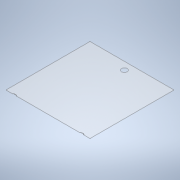
# Autodesk Inventor part: porta
Saved by Autodesk Inventor 2022 (Build 260153000, 153)
## iProperties
Created: 2022-02-18
Part Number: porta
Material: Acrílico
Document SubType Name: Modeling
Designer: mathe
Density: 1.188 g/cm^3
Appearance: Transparente - Claro
Author: mathe
Autodesk Inventor part; units mm, degrees
ref_plane "YZ Plane" through (0, 0, 0) normal (1, 0, 0) x (0, 1, 0)
ref_plane "XZ Plane" through (0, 0, 0) normal (0, 1, 0) x (-1, 0, 0)
ref_plane "XY Plane" through (0, 0, 0) normal (0, 0, 1) x (1, 0, 0)
sketch "Esboço1" plane through (0, 0, 0) normal (0, 1, 0) x (-1, 0, 0)
  line L0 (0, 0) -> (440, 0)
  line L1 (440, 0) -> (440, -440)
  line L2 (440, -440) -> (0, -440)
  line L3 (0, -440) -> (0, 0)
  dimension "d0" = 440
  dimension "d1" = 440
  constraints: 8 end point, 2 parallel, 1 horizontal, 1 perpendicular
  measures "d0" distance of L1.end L2.end
  measures "d1" distance of L0.end L1.end
extrude "Extrusão1" add sketch "Esboço1" along normal blind 2
sketch "Esboço2" plane through (0, 2, 0) normal (0, 1, 0) x (1, 0, 0)
  point P0 (0, 0)
  point P1 (-40, 5)
  point P2 (-47, 5)
  point P3 (-400, 5)
  point P4 (-393, 5)
hole "Furo1" at (-40, 2, -5) at (-47, 2, -5) at (-400, 2, -5) at (-393, 2, -5) direction (0, -1, 0) diameter 2 end through all
fillet "Arredondamento1" radius 2 4 edges at (0, 1, -440) (-440, 1, -440) (-440, 1, 0) (0, 1, 0)
sketch "Esboço3" plane through (0, 2, 0) normal (0, 1, 0) x (1, 0, 0)
  point P0 (0, 0)
  point P1 (-220, 400)
hole "Furo2" at (-220, 2, -400) direction (0, -1, 0) diameter 30 end through all
sketch "Esboço4" plane through (0, 2, 0) normal (0, 1, 0) x (1, 0, 0)
  line L0 (-438, 0) -> (-2, 0) projected
  line L1 (-34.0574, 0) -> (-52.0574, 0)
  line L2 (-52.0574, 0) -> (-52.0574, 3)
  line L3 (-52.0574, 3) -> (-34.0574, 3)
  line L4 (-34.0574, 3) -> (-34.0574, 0)
  line L5 (-387.0061, 0) -> (-405.0061, 0)
  line L6 (-405.0061, 0) -> (-405.0061, 3)
  line L7 (-405.0061, 3) -> (-387.0061, 3)
  line L8 (-387.0061, 3) -> (-387.0061, 0)
  point P0 (0, 0)
  dimension "d19" = 18
  dimension "d20" = 3
  dimension "d21" = 18
  dimension "d22" = 3
  constraints: 16 end point, 4 parallel, 2 horizontal, 2 perpendicular
  measures "d19" distance of L2.end L3.end
  measures "d20" distance of L1.end L2.end
  measures "d21" distance of L6.end L7.end
  measures "d22" distance of L5.end L6.end
extrude "Extrusão2" cut sketch "Esboço4" against normal blind 2
